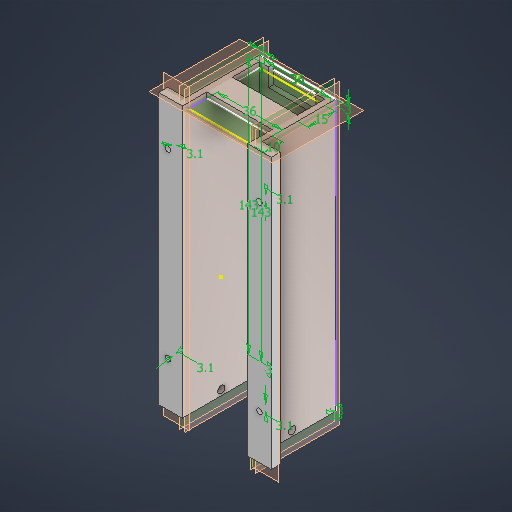
# Autodesk Inventor part: suport_batterie
Saved by Autodesk Inventor 2026.1 (Build 301233000, 233)
## iProperties
Created: 2026-03-03
Part Number: suport_batterie
Material: Generic
Document SubType Name: Modeling
Designer: fheli
Density: 1 g/cm^3
Appearance: Default
Author: fheli
Autodesk Inventor part; units mm, degrees
ref_plane "YZ Plane" through (0, 0, 0) normal (1, 0, 0) x (0, 1, 0)
ref_plane "XZ Plane" through (0, 0, 0) normal (0, 1, 0) x (-1, 0, 0)
ref_plane "XY Plane" through (0, 0, 0) normal (0, 0, 1) x (1, 0, 0)
sketch "Sketch1" plane through (0, 0, 0) normal (0, 0, 1) x (1, 0, 0)
  line L0 (18, -71.5) -> (-18, -71.5)
  line L1 (-18, -71.5) -> (-18, 71.5)
  line L2 (-18, 71.5) -> (18, 71.5)
  line L3 (18, 71.5) -> (18, -71.5)
  line L4 (18, -71.5) -> (-18, 71.5) construction
  line L5 (-18, -71.5) -> (18, 71.5) construction
  line L6 (18, -71.5) -> (21, -71.5)
  line L7 (21, -71.5) -> (21, 71.5)
  line L8 (21, 71.5) -> (18, 71.5)
  line L9 (18, 71.5) -> (18, -71.5)
  line L10 (-18, -71.5) -> (-21, -71.5)
  line L11 (-21, -71.5) -> (-21, 71.5)
  line L12 (-21, 71.5) -> (-18, 71.5)
  line L13 (-18, 71.5) -> (-18, -71.5)
  line L14 (-21, 71.5) -> (21, 71.5)
  line L15 (21, 71.5) -> (21, 74.5)
  line L16 (21, 74.5) -> (-21, 74.5)
  line L17 (-21, 74.5) -> (-21, 71.5)
  line L18 (-21, -71.5) -> (-18, -71.5)
  line L19 (-18, -71.5) -> (-18, -74.5)
  line L20 (-18, -74.5) -> (-21, -74.5)
  line L21 (-21, -74.5) -> (-21, -71.5)
  line L22 (18, -71.5) -> (21, -71.5)
  line L23 (21, -71.5) -> (21, -74.5)
  line L24 (21, -74.5) -> (18, -74.5)
  line L25 (18, -74.5) -> (18, -71.5)
  point P0 (0, 0)
  dimension "d0" = 36
  dimension "d1" = 143
  dimension "d3" = 3
  dimension "d4" = 143
  dimension "d5" = 3
  dimension "d6" = 3
  dimension "d7" = 3
  dimension "d8" = 3
  constraints: 52 end point, 12 parallel, 6 horizontal, 6 perpendicular, 2 midpoint
  measures "d0" distance of L1.end L2.end
  measures "d1" distance of L0.end L1.end
  measures "d3" distance of L11.end L12.end
  measures "d4" distance of L10.end L11.end
  measures "d5" distance of L15.end L14.end
  measures "d6" distance of L18.end L19.end
  measures "d7" distance of L23.end L24.end
  measures "d8" distance of L22.end L23.end
extrude "Extrusion1" add sketch "Sketch1" along normal blind 3 contours L0 L1 L2 L3
extrude "Extrusion2" add sketch "Sketch1" along normal blind 42 contours L3 L8 L7 L6 | L6 L23 L24 L25 | L10 L11 L12 L1 | L19 L20 L21 L10 | L2 L12 L17 L16 L15 L8
ref_plane "Work Plane1" through (-18, 73, 3) normal (0, -1, 0) x (1, 0, 0)
sketch "Sketch2" plane through (-18, 71.5, 3) normal (0, -1, 0) x (1, 0, 0)
  point P0 (18, -3)
ref_plane "Work Plane2" through (-18, 71.5, 3) normal (0, -1, 0) x (1, 0, 0)
sketch "Sketch3" plane through (-18, 71.5, 3) normal (0, -1, 0) x (1, 0, 0)
  line L0 (0, 0) -> (36, 0) projected
  line L1 (36, -3) -> (36, 39) projected
  line L2 (0, 0) -> (36, 0)
  line L3 (36, 0) -> (36, 15)
  line L4 (36, 15) -> (0, 15)
  line L5 (0, 15) -> (0, 0)
  line L6 (39, 39) -> (-3, 39) projected
  line L7 (0, 39) -> (36, 39)
  line L8 (36, 39) -> (36, 29)
  line L9 (36, 29) -> (0, 29)
  line L10 (0, 29) -> (0, 39)
  point P0 (18, -3)
  dimension "d14" = 15
  dimension "d15" = 36
  dimension "d16" = 10
  constraints: 16 end point, 4 parallel, 2 horizontal, 2 perpendicular, 2 point on line
  measures "d14" distance of L3.end L2.end
  measures "d15" distance of L8.end L9.end
  measures "d16" distance of L7.end L8.end
extrude "Extrusion3" cut sketch "Sketch3" against normal blind 42 contours L5 L4 L1 L0
extrude "Extrusion4" cut sketch "Sketch3" against normal blind 42 contours L9 L10 L6 L1
ref_plane "Work Plane3" through (-21, -74.5, 0) normal (-1, 0, 0) x (0, 0, 1)
sketch "Sketch4" plane through (-21, -74.5, 0) normal (-1, 0, 0) x (0, 0, 1)
  line L0 (42, 149) -> (42, 0) projected
  line L1 (32, 149) -> (42, 149) projected
  line L2 (42, 0) -> (37, 0)
  line L3 (37, 0) -> (37, 149)
  line L4 (37, 149) -> (42, 149)
  line L5 (42, 149) -> (42, 0)
  point P0 (0, 74.5)
  dimension "d22" = 5
  constraints: 8 end point, 2 parallel, 1 horizontal, 1 midpoint, 1 perpendicular
  measures "d22" distance of L3.end L4.end
extrude "Extrusion5" add sketch "Sketch4" along normal blind 10
ref_plane "Work Plane4" through (21, -74.5, 0) normal (1, 0, 0) x (0, 0, -1)
sketch "Sketch5" plane through (21, -74.5, 0) normal (1, 0, 0) x (0, 0, -1)
  line L0 (0, 149) -> (-42, 149) projected
  line L1 (-42, 149) -> (-37, 149)
  line L2 (-37, 149) -> (-37, 0)
  line L3 (-37, 0) -> (-42, 0)
  line L4 (-42, 0) -> (-42, 149)
  point P0 (0, 74.5)
  dimension "d26" = 5
  dimension "d27" = 149
  constraints: 8 end point, 2 parallel, 1 horizontal, 1 perpendicular
  measures "d26" distance of L2.end L3.end
  measures "d27" distance of L1.end L2.end
extrude "Extrusion6" add sketch "Sketch5" along normal blind 10
ref_plane "Work Plane5" through (0, 0, 42) normal (0, 0, 1) x (1, 0, 0)
sketch "Sketch6" plane through (0, 0, 42) normal (0, 0, 1) x (1, 0, 0)
  circle A0 centre (-26, -50) radius 1.55
  circle A1 centre (-26, 50) radius 1.55
  point P0 (0, 0)
  dimension "d31" = 3.1
  dimension "d32" = 3.1
  constraints: 2 centre point
  measures "d31" diameter of A0
  measures "d32" diameter of A1
ref_plane "Work Plane6" through (0, 0, 42) normal (0, 0, 1) x (1, 0, 0)
sketch "Sketch7" plane through (0, 0, 42) normal (0, 0, 1) x (1, 0, 0)
  circle A0 centre (24.5, -50) radius 1.55
  circle A1 centre (24.5, 50) radius 1.55
  point P0 (0, 0)
  dimension "d34" = 3.1
  dimension "d35" = 3.1
  constraints: 2 centre point
  measures "d34" diameter of A0
  measures "d35" diameter of A1
extrude "Extrusion7" cut sketch "Sketch6" against normal blind 10 contours A0
extrude "Extrusion8" cut sketch "Sketch7" against normal blind 10 contours A0
extrude "Extrusion9" cut sketch "Sketch6" against normal blind 10 contours A1
extrude "Extrusion10" cut sketch "Sketch7" against normal blind 10 contours A1
ref_plane "Work Plane7" through (-18, -74.5, 42) normal (1, 0, 0) x (0, 0, -1)
sketch "Sketch8" plane through (-18, -74.5, 42) normal (1, 0, 0) x (0, 0, -1)
  circle A0 centre (18, 3) radius 2
  point P0 (42, 74.5)
  dimension "d45" = 4
  constraints: 1 centre point
  measures "d45" diameter of A0
ref_plane "Work Plane8" through (18, -74.5, 42) normal (-1, 0, 0) x (0, 0, 1)
sketch "Sketch9" plane through (18, -74.5, 42) normal (-1, 0, 0) x (0, 0, 1)
  circle A0 centre (-18, 3) radius 2
  point P0 (-42, 74.5)
  dimension "d47" = 4
  constraints: 1 centre point
  measures "d47" diameter of A0
extrude "Extrusion11" cut sketch "Sketch8" against normal blind 10
extrude "Extrusion12" cut sketch "Sketch9" against normal blind 10
move faces "Move1" translate (0, 0, 3.5) faces at (-20.15, -16.6667, 42)
move faces "Move2" translate (0, 0, 3.5) faces at (-22.15, -16.6667, 37)
move faces "Move3" translate (0, 0, 3.5) faces at (29.335, 16.543, 42)
move faces "Move4" translate (0, 0, 3.5) faces at (29.335, -16.543, 37)
sketch "Sketch10" plane through (-21, 74.5, 0) normal (0, 1, 0) x (1, 0, 0)
  point P0 (21, 0)
ref_plane "Work Plane9" through (-21, 74.5, 0) normal (0, 1, 0) x (1, 0, 0)
sketch "Sketch11" plane through (-21, 74.5, 0) normal (0, 1, 0) x (1, 0, 0)
  line L0 (42, 0) -> (0, 0) projected
  line L1 (34, -3) -> (8, -3)
  line L2 (8, -3) -> (8, 0)
  line L3 (8, 0) -> (34, 0)
  line L4 (34, 0) -> (34, -3)
  point P0 (21, 0)
  dimension "d65" = 26
  constraints: 8 end point, 2 parallel, 1 horizontal, 1 perpendicular, 1 point on line
  measures "d65" distance of L2.end L3.end
extrude "Extrusion13" cut sketch "Sketch11" against normal blind 10
body "Solid1"
